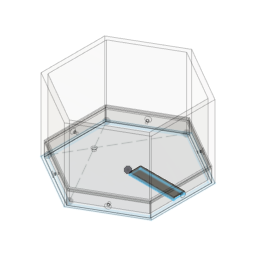
Hexashelf (Autodesk Fusion 360 design; units mm, degrees)
Autodesk Fusion 360 part; units mm, degrees
sketch "Sketch1" plane through (0, 0, 0) normal (0, 0, 1) x (1, 0, 0) in component "Shelf"
  line L0 (0, 0) -> (80, 0)
  line L1 (80, 0) -> (120, 69.282)
  line L2 (120, 69.282) -> (80, 138.5641)
  line L3 (80, 138.5641) -> (0, 138.5641)
  line L4 (0, 138.5641) -> (-40, 69.282)
  line L5 (-40, 69.282) -> (0, 0)
  line L6 (123.1384, 69.282) -> (81.5692, 141.282)
  line L7 (81.5692, 141.282) -> (-1.5692, 141.282)
  line L8 (-1.5692, 141.282) -> (-43.1384, 69.282)
  line L9 (-43.1384, 69.282) -> (-1.5692, -2.718)
  line L10 (-1.5692, -2.718) -> (81.5692, -2.718)
  line L11 (81.5692, -2.718) -> (123.1384, 69.282)
  line L12 (1.3175, 2.282) -> (78.6825, 2.282)
  line L13 (78.6825, 2.282) -> (117.3649, 69.282)
  line L14 (117.3649, 69.282) -> (78.6825, 136.282)
  line L15 (78.6825, 136.282) -> (1.3175, 136.282)
  line L16 (1.3175, 136.282) -> (-37.3649, 69.282)
  line L17 (-37.3649, 69.282) -> (1.3175, 2.282)
  point P0 (40, 69.282)
  point P1 (40, 69.282)
  point P2 (40, 69.282)
  dimension "d1" = 80
  dimension "d2" = 72
  dimension "d3" = 67
  constraint coincident L0.start L5.end
  constraint coincident P2 P1
  measures "d1" distance of L0.start L0.end
  measures "d2" distance of P2 L11
  measures "d3" distance of P2 L17
extrude "Extrude1" add sketch "Sketch1" along normal blind 80 contours L12 L13 L14 L15 L16 L17 makes body 1 in component "Shelf"
extrude "Extrude2" add sketch "Sketch1" along normal blind 100 contours L0 L1 L2 L3 L4 L5 | L6 L7 L8 L9 L10 L11 bodies 1 in component "Shelf"
sketch "Sketch1 (2)" plane through (0, 0, 80) normal (0, 0, 1) x (-1, 0, 0) in component "Diffuser"
  line L0 (37.3649, -69.282) -> (-1.3175, -2.282)
  line L1 (-1.3175, -2.282) -> (-78.6825, -2.282)
  line L2 (-78.6825, -2.282) -> (-117.3649, -69.282)
  line L3 (-117.3649, -69.282) -> (-78.6825, -136.282)
  line L4 (-78.6825, -136.282) -> (-1.3175, -136.282)
  line L5 (-1.3175, -136.282) -> (37.3649, -69.282)
  line L6 (-116.9726, -69.3148) -> (-78.5212, -136.0482)
  line L7 (-78.5212, -136.0482) -> (-1.5027, -136.115)
  line L8 (-1.5027, -136.115) -> (37.0644, -69.4484)
  line L9 (37.0644, -69.4484) -> (-1.387, -2.715)
  line L10 (-1.387, -2.715) -> (-78.4055, -2.6482)
  line L11 (-78.4055, -2.6482) -> (-116.9726, -69.3148)
  point P0 (-39.9541, -69.3816)
  dimension "d9" = 66.7
  measures "d9" distance of P0 L11
extrude "Extrude1'" add sketch "Sketch1 (2)" along normal blind 3 separate body contours L6 L7 L8 L9 L10 L11 makes body 2 in component "Diffuser"
sketch "Sketch1 (3)" plane through (0, 0, 83) normal (0, 0, 1) x (-1, 0, 0) in component "Base"
  line L0 (-78.4055, -2.6482) -> (-116.9726, -69.3148)
  line L1 (-116.9726, -69.3148) -> (-78.5212, -136.0482)
  line L2 (-78.5212, -136.0482) -> (-1.5027, -136.115)
  line L3 (-1.5027, -136.115) -> (37.0644, -69.4484)
  line L4 (37.0644, -69.4484) -> (-1.387, -2.715)
  line L5 (-1.387, -2.715) -> (-78.4055, -2.6482)
  line L6 (2.1228, -211.5233) -> (64.2459, -103.9233)
  line L7 (64.2459, -103.9233) -> (2.1231, 3.6767)
  line L8 (2.1231, 3.6767) -> (-122.1227, 3.6769)
  line L9 (-122.1227, 3.6769) -> (-184.2457, -103.923)
  line L10 (-184.2457, -103.923) -> (-122.1229, -211.5231)
  line L11 (-122.1229, -211.5231) -> (2.1228, -211.5233)
  line L12 (-120.0445, -207.9231) -> (0.0444, -207.9233)
  line L13 (0.0444, -207.9233) -> (60.089, -103.9233)
  line L14 (60.089, -103.9233) -> (0.0447, 0.0767)
  line L15 (0.0447, 0.0767) -> (-120.0442, 0.0769)
  line L16 (-120.0442, 0.0769) -> (-180.0888, -103.923)
  line L17 (-180.0888, -103.923) -> (-120.0445, -207.9231)
  point P0 (-59.9999, -103.9232)
  point P1 (-59.9999, -103.9232)
  dimension "d12" = 107.6
  dimension "d13" = 104
  constraint coincident P1 P0
  measures "d12" distance of P1 L11
  measures "d13" distance of P1 L17
extrude "Extrude1''" add sketch "Sketch1 (3)" along normal blind 17 separate body contours L6 L7 L8 L9 L10 L11 makes body 3 in component "Base"
extrude "Extrude2'" add sketch "Sketch1 (3)" along normal blind 17 contours L0 L1 L2 L3 L4 L5 | L12 L13 L14 L15 L16 L17 bodies 3 in component "Base"
extrude "Extrude3" cut sketch "Sketch1 (3)" along normal blind 14 contours L0 L1 L2 L3 L4 L5 | L12 L13 L14 L15 L16 L17 bodies 3 in component "Base"
sketch "Sketch2" plane through (0, 141.282, 0) normal (0, 1, 0) x (-1, 0, 0) in component "Shelf"
  line L0 (-81.5692, 0) -> (1.5692, 0)
  line L1 (1.5692, 0) -> (1.5692, 100)
  line L2 (1.5692, 100) -> (-81.5692, 100)
  line L3 (-81.5692, 100) -> (-81.5692, 0)
  line L4 (-81.5692, 100) -> (1.5692, 86.3693) construction
  line L5 (1.5692, 100) -> (-81.5692, 83.3017) construction
  constraint coincident L2.end L3.start
  constraint coincident L1 L4.end
  constraint coincident L1.end L2.start
  constraint coincident L3 L5.end
sketch "Sketch3" plane through (-62.3538, 36, 0) normal (-0.866025, 0.5, 0) x (-0.5, -0.866025, 0) in component "Shelf"
  line L0 (-121.5692, 0) -> (-38.4308, 0)
  line L1 (-38.4308, 0) -> (-38.4308, 100)
  line L2 (-38.4308, 100) -> (-121.5692, 100)
  line L3 (-121.5692, 100) -> (-121.5692, 0)
  line L4 (-121.5692, 100) -> (-38.4308, 87.4373) construction
  line L5 (-38.4308, 100) -> (-121.5692, 83.6489) construction
  constraint coincident L2.end L3.start
  constraint coincident L1 L4.end
  constraint coincident L1.end L2.start
  constraint coincident L3 L5.end
sketch "Sketch4" plane through (122.3538, 70.641, 0) normal (0.866025, 0.5, 0) x (-0.5, 0.866025, 0) in component "Shelf"
  line L0 (-1.5692, 0) -> (81.5692, 0)
  line L1 (81.5692, 0) -> (81.5692, 100)
  line L2 (81.5692, 100) -> (-1.5692, 100)
  line L3 (-1.5692, 100) -> (-1.5692, 0)
  line L4 (81.5692, 100) -> (-1.5692, 86.4283) construction
  line L5 (-1.5692, 100) -> (81.5692, 83.3738) construction
  constraint coincident L1.end L2.start
  constraint coincident L3 L4.end
  constraint coincident L2.end L3.start
  constraint coincident L1 L5.end
hole "Hole1" at (102.3538, 105.2821, 91.5371) direction (-0.866025, -0.5, 0) diameter 3 depth 224 tip angle 180 bodies 3 in component "Base"
hole "Hole1'" at (102.3538, 105.2821, 91.5371) direction (-0.866025, -0.5, 0) diameter 3 depth 224 tip angle 180 bodies 1 in component "Shelf"
hole "Hole2" at (40, 141.282, 91.4996) direction (0, -1, 0) diameter 3 depth 224 tip angle 180 bodies 3 in component "Base"
hole "Hole2'" at (40, 141.282, 91.4996) direction (0, -1, 0) diameter 3 depth 224 tip angle 180 bodies 1 in component "Shelf"
hole "Hole3" at (-22.3538, 105.2821, 91.5706) direction (0.866025, -0.5, 0) diameter 3 depth 224 tip angle 180 bodies 3 in component "Base"
hole "Hole3'" at (-22.3538, 105.2821, 91.5706) direction (0.866025, -0.5, 0) diameter 3 depth 224 tip angle 180 bodies 1 in component "Shelf"
chamfer "Chamfer2" distance 3 angle 45 6 edges at (103.053, 104.071, 92.0795) (103.0531, 34.4933, 91.0282) (39.4575, -2.718, 90.1011) (-21.6546, 32.071, 90.9947) (-21.6545, 106.4933, 92.113) (40.5424, 141.282, 90.1011) on bodies 1 in component "Shelf"
sketch "Sketch2 (2)" plane through (0, 0, 83) normal (0, 0, 1) x (-1, 0, 0) in component "Base"
  line L0 (-180, -105) -> (0, -208) construction
  line L1 (-120, -208) -> (60, -105) construction
hole "Hole4" at (59.9999, 173.6666, 97) direction (0, 0, 1) diameter 4 depth 5 tip angle 180 bodies 3 in component "Base"
chamfer "Chamfer1" distance 1 angle 45 1 edges at (61.8646, 174.3899, 97) on bodies 3 in component "Base"
sketch "Sketch1 (4)" plane through (0, 0, 0) normal (0, 0, 1) x (1, 0, 0) in component "Base (1)"
  line L0 (70, 40.4145) -> (0, 80.829)
  line L1 (0, 80.829) -> (-70, 40.4145)
  line L2 (-70, 40.4145) -> (-70, -40.4145)
  line L3 (-70, -40.4145) -> (0, -80.829)
  line L4 (0, -80.829) -> (70, -40.4145)
  line L5 (70, -40.4145) -> (70, 40.4145)
  line L6 (73, 42.1466) -> (0, 84.2931)
  line L7 (0, 84.2931) -> (-73, 42.1466)
  line L8 (-73, 42.1466) -> (-73, -42.1466)
  line L9 (-73, -42.1466) -> (0, -84.2931)
  line L10 (0, -84.2931) -> (73, -42.1466)
  line L11 (73, -42.1466) -> (73, 42.1466)
  line L12 (76, 43.8786) -> (0, 87.7572)
  line L13 (0, 87.7572) -> (-76, 43.8786)
  line L14 (-76, 43.8786) -> (-76, -43.8786)
  line L15 (-76, -43.8786) -> (0, -87.7572)
  line L16 (0, -87.7572) -> (76, -43.8786)
  line L17 (76, -43.8786) -> (76, 43.8786)
extrude "Extrude1'''" add sketch "Sketch1 (4)" along normal blind 3 separate body contours L0 L1 L2 L3 L4 L5 | L6 L7 L8 L9 L10 L11 makes body 4 in component "Base (1)"
extrude "Extrude2''" add sketch "Sketch1 (4)" along normal blind 17 contours L6 L7 L8 L9 L10 L11 bodies 4 in component "Base (1)"
sketch "Sketch1 (5)" plane through (0, 0, 0) normal (0, 0, 1) x (1, 0, 0) in component "Shelf (1)"
  line L0 (-76, -43.8786) -> (0, -87.7572)
  line L1 (0, -87.7572) -> (76, -43.8786)
  line L2 (76, -43.8786) -> (76, 43.8786)
  line L3 (76, 43.8786) -> (0, 87.7572)
  line L4 (0, 87.7572) -> (-76, 43.8786)
  line L5 (-76, 43.8786) -> (-76, -43.8786)
  line L6 (-73.3, -42.3198) -> (0, -84.6395)
  line L7 (0, -84.6395) -> (73.3, -42.3198)
  line L8 (73.3, -42.3198) -> (73.3, 42.3198)
  line L9 (73.3, 42.3198) -> (0, 84.6395)
  line L10 (0, 84.6395) -> (-73.3, 42.3198)
  line L11 (-73.3, 42.3198) -> (-73.3, -42.3198)
  line L12 (70, 40.4145) -> (0, 80.829)
  line L13 (0, 80.829) -> (-70, 40.4145)
  line L14 (-70, 40.4145) -> (-70, -40.4145)
  line L15 (-70, -40.4145) -> (0, -80.829)
  line L16 (0, -80.829) -> (70, -40.4145)
  line L17 (70, -40.4145) -> (70, 40.4145)
  dimension "d47" = 73.3
  measures "d47" distance of origin L11
extrude "Extrude1''''" add sketch "Sketch1 (5)" along normal blind 100 separate body contours L0 L1 L2 L3 L4 L5 | L6 L7 L8 L9 L10 L11 makes body 5 in component "Shelf (1)"
extrude "Extrude2'''" cut sketch "Sketch1 (5)" along normal blind 20 contours L6 L7 L8 L9 L10 L11 bodies 5 in component "Shelf (1)"
sketch "Sketch2 (3)" plane through (76, 0, 0) normal (1, 0, 0) x (0, 1, 0) in component "Shelf (1)"
  line L0 (-43.8786, 0) -> (43.8786, 0)
  line L1 (43.8786, 0) -> (43.8786, 100)
  line L2 (43.8786, 100) -> (-43.8786, 100)
  line L3 (-43.8786, 100) -> (-43.8786, 0)
  line L4 (-43.8786, 0) -> (43.8786, 16.9474) construction
  line L5 (43.8786, 0) -> (-43.8786, 16.9474) construction
  constraint coincident L0.start L3.end
  constraint coincident L1 L4.end
  constraint coincident L0.end L1.start
  constraint coincident L3 L5.end
sketch "Sketch4 (2)" plane through (38, 65.8179, 0) normal (0.5, 0.866025, 0) x (-0.866025, 0.5, 0) in component "Shelf (1)"
  line L0 (-43.8786, 0) -> (43.8786, 0)
  line L1 (43.8786, 0) -> (43.8786, 100)
  line L2 (43.8786, 100) -> (-43.8786, 100)
  line L3 (-43.8786, 100) -> (-43.8786, 0)
  line L4 (-43.8786, 0) -> (43.8786, 17.0002) construction
  line L5 (43.8786, 0) -> (-43.8786, 17.0002) construction
  constraint coincident L0.start L3.end
  constraint coincident L1 L4.end
  constraint coincident L0.end L1.start
  constraint coincident L3 L5.end
sketch "Sketch5" plane through (38, -65.8179, 0) normal (0.5, -0.866025, 0) x (0.866025, 0.5, 0) in component "Shelf (1)"
  line L0 (-43.8786, 0) -> (43.8786, 0)
  line L1 (43.8786, 0) -> (43.8786, 100)
  line L2 (43.8786, 100) -> (-43.8786, 100)
  line L3 (-43.8786, 100) -> (-43.8786, 0)
  line L4 (44, 17) -> (-43.8786, 0) construction
  line L5 (43.8786, 0) -> (-43.8786, 17) construction
  constraint coincident L0.start L3.end
  constraint coincident L0.end L1.start
  constraint coincident L3 L5.end
hole "Hole1''" at (76, -0.0002, 8.4737) direction (-1, 0, 0) diameter 3 depth 200 tip angle 180 bodies 4 in component "Base (1)"
hole "Hole1'''" at (76, -0.0002, 8.4737) direction (-1, 0, 0) diameter 3 depth 200 tip angle 180 bodies 5 in component "Shelf (1)"
hole "Hole2''" at (38.0003, 65.8177, 8.5002) direction (-0.5, -0.866025, 0) diameter 3 depth 200 tip angle 180 bodies 4 in component "Base (1)"
hole "Hole2'''" at (38.0003, 65.8177, 8.5002) direction (-0.5, -0.866025, 0) diameter 3 depth 200 tip angle 180 bodies 5 in component "Shelf (1)"
hole "Hole3''" at (38.0262, -65.8028, 8.4941) direction (-0.5, 0.866025, 0) diameter 3 depth 200 tip angle 180 bodies 4 in component "Base (1)"
hole "Hole3'''" at (38.0262, -65.8028, 8.4941) direction (-0.5, 0.866025, 0) diameter 3 depth 200 tip angle 180 bodies 5 in component "Shelf (1)"
chamfer "Chamfer1'" distance 2 angle 45 6 edges at (38.4959, -65.5316, 9.8926) (-38.4694, -65.5469, 7.1017) (76, -1.3986, 9.0162) (38.4701, 65.5465, 7.1017) (-38.4436, 65.5618, 9.8926) (-76, -1.3986, 7.9313) on bodies 5 in component "Shelf (1)"
sketch "Sketch1 (6)" plane through (0, 0, 3) normal (0, 0, 1) x (-1, 0, 0) in component "Hexashelf v2"
  line L0 (-70, -40.4145) -> (0, -80.829)
  line L1 (0, -80.829) -> (70, -40.4145)
  line L2 (70, -40.4145) -> (70, 40.4145)
  line L3 (70, 40.4145) -> (0, 80.829)
  line L4 (0, 80.829) -> (-70, 40.4145)
  line L5 (-70, 40.4145) -> (-70, -40.4145)
  line L6 (0, 80.829) -> (70, -40.4145) construction
  line L7 (70, 40.4145) -> (0, -80.829) construction
  constraint coincident L3.end L4.start
  constraint coincident L1.end L2.start
  constraint coincident L2.end L3.start
  constraint coincident L0.end L1.start
hole "Hole4'" at (-46.6666, 0.0001, 3) direction (0, 0, -1) diameter 4.5 depth 5 tip angle 180 bodies 4 in component "Base (1)"
chamfer "Chamfer1''" distance 1 angle 45 1 edges at (-48.7644, 0.8137, 3) on bodies 4 in component "Base (1)"
sketch "Sketch1 (7)" plane through (0, 0, 17) normal (0, 0, 1) x (-1, 0, 0) in component "Glass"
  line L0 (-70, -40.4145) -> (-70, 40.4145)
  line L1 (-70, 40.4145) -> (0, 80.829)
  line L2 (0, 80.829) -> (70, 40.4145)
  line L3 (70, 40.4145) -> (70, -40.4145)
  line L4 (70, -40.4145) -> (0, -80.829)
  line L5 (0, -80.829) -> (-70, -40.4145)
  line L6 (-73, 42.1466) -> (-73, -42.1466)
  line L7 (-73, -42.1466) -> (0, -84.2931)
  line L8 (0, -84.2931) -> (73, -42.1466)
  line L9 (73, -42.1466) -> (73, 42.1466)
  line L10 (73, 42.1466) -> (0, 84.2931)
  line L11 (0, 84.2931) -> (-73, 42.1466)
  line L12 (-72, -41.5692) -> (0, -83.1384)
  line L13 (0, -83.1384) -> (72, -41.5692)
  line L14 (72, -41.5692) -> (72, 41.5692)
  line L15 (72, 41.5692) -> (0, 83.1384)
  line L16 (0, 83.1384) -> (-72, 41.5692)
  line L17 (-72, 41.5692) -> (-72, -41.5692)
  dimension "d75" = 72
  measures "d75" distance of origin L17
extrude "Extrude1'''''" add sketch "Sketch1 (7)" along normal blind 3 separate body contours L0 L1 L2 L3 L4 L5 | L12 L13 L14 L15 L16 L17 makes body 6 in component "Glass"
sketch "Sketch1 (8)" plane through (0, 0, 3) normal (0, 0, 1) x (1, 0, 0) in component "Cable-Cover"
  line L0 (70, 7.5) -> (10, 7.5)
  line L1 (10, 7.5) -> (10, -7.5)
  line L2 (10, -7.5) -> (70, -7.5)
  line L3 (70, -7.5) -> (70, 7.5)
  line L4 (70, 7.5) -> (10, 7.5)
  line L5 (10, 7.5) -> (10, 6)
  line L6 (10, 6) -> (70, 6)
  line L7 (70, 6) -> (70, 7.5)
  line L8 (70, -7.5) -> (10, -7.5)
  line L9 (10, -7.5) -> (10, -6)
  line L10 (10, -6) -> (70, -6)
  line L11 (70, -6) -> (70, -7.5)
  dimension "d78" = 60
  dimension "d79" = 15
  constraint horizontal L0
  constraint vertical L1
  constraint horizontal L2
  constraint vertical L3
  constraint horizontal L4
  constraint vertical L5
  constraint horizontal L6
  constraint vertical L7
  constraint coincident L1 L5.end
  constraint horizontal L8
  constraint vertical L9
  constraint horizontal L10
  constraint vertical L11
  constraint coincident L1 L9.end
  measures "d78" distance of L0.start L0.end
  measures "d79" distance of L0.start L2.end
extrude "Extrude1''''''" add sketch "Sketch1 (8)" along normal blind 3 separate body makes body 7 in component "Cable-Cover"
extrude "Extrude2''''" cut sketch "Sketch1 (8)" along normal blind 2 contours L1 L3 L6 L10 bodies 7 in component "Cable-Cover"
component "Hexashelf" placed x (1, 0, 0) y (0, 1, 0) z (0, 0, 1) at (0, 0, 0)
component "Hexashelf v2" placed x (1, 0, 0) y (0, 1, 0) z (0, 0, 1) at (0, 0, 0)
component "Base" placed x (1, 0, 0) y (0, 1, 0) z (0, 0, 1) at (0, 0, 0) in component "Hexashelf"
component "Diffuser" placed x (1, 0, 0) y (0, 1, 0) z (0, 0, 1) at (0, 0, 0) in component "Hexashelf"
component "Shelf" placed x (1, 0, 0) y (0, 1, 0) z (0, 0, 1) at (0, 0, 0) in component "Hexashelf"
component "Base (1)" placed x (1, 0, 0) y (0, 1, 0) z (0, 0, 1) at (0, 0, 0) in component "Hexashelf v2"
component "Shelf (1)" placed x (1, 0, 0) y (0, 1, 0) z (0, 0, 1) at (0, 0, 0) in component "Hexashelf v2"
component "Glass" placed x (1, 0, 0) y (0, 1, 0) z (0, 0, 1) at (0, 0, 0) in component "Hexashelf v2"
component "Cable-Cover" placed x (1, 0, 0) y (0, 1, 0) z (0, 0, 1) at (0, 0, 0) in component "Hexashelf v2"
